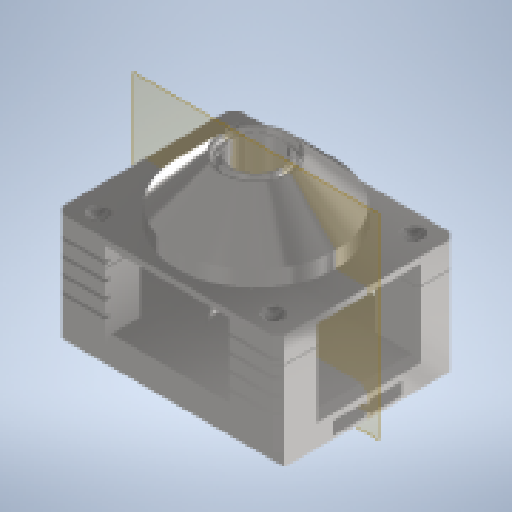
# Autodesk Inventor part: robotic-arm_base
Saved by Autodesk Inventor 2023 (Build 270158000, 158)
## iProperties
Created: 2023-11-19
Part Number: robotic-arm_base
Material: Steel, Mild
Document SubType Name: Modeling
Designer: Beatrice
Density: 7.85 g/cm^3
Appearance: Semi-Polished
Author: Beatrice
Autodesk Inventor part; units mm, degrees
ref_plane "YZ Plane" through (0, 0, 0) normal (1, 0, 0) x (0, 1, 0)
ref_plane "XZ Plane" through (0, 0, 0) normal (0, 1, 0) x (-1, 0, 0)
ref_plane "XY Plane" through (0, 0, 0) normal (0, 0, 1) x (1, 0, 0)
sketch "Sketch1" plane through (0, 0, 0) normal (1, 0, 0) x (0, 1, 0)
  line L0 (0, 25.2) -> (0, -4.2) construction
  line L1 (-30, 0) -> (5, 0) construction
  line L2 (0, 0) -> (-25, 0)
  line L3 (-25, 7) -> (-25, 0)
  line L4 (-7.6, 21) -> (-7.6, 6)
  line L5 (-7.6, 6) -> (0, 6)
  line L6 (0, 6) -> (0, 0)
  line L7 (-25, 7) -> (-11, 21)
  line L8 (-11, 21) -> (-7.6, 21)
  line L9 (-10.3, 21) -> (-8.3, 21)
  line L10 (-8.3, 21) -> (-8.3, 19)
  line L11 (-8.3, 19) -> (-10.3, 19)
  line L12 (-10.3, 19) -> (-10.3, 21)
  point P0 (-3.8, 6)
  point P1 (-9.3, 21)
  point P2 (-9.3, 19)
  dimension "d3" = 7.6
  dimension "d4" = 25
  dimension "d6" = 6
  dimension "d7" = 135
  dimension "d67" = 15
  dimension "d68" = 2
  constraints: 22 end point, 4 perpendicular, 3 midpoint, 3 point on line, 2 parallel, 1 collinear, 1 horizontal, 1 vertical alignment
  measures "d3" distance between parallel lines of L0 L4
  measures "d4" distance of L2.end L2.start
  measures "d6" distance between parallel lines of L5 L2
  measures "d7" angle of L3 L7
  measures "d67" vertical distance of point (-3.8, 6) point (-9.3, 21)
  measures "d68" distance of L10.end L11.end
revolve "Revolution1" add sketch "Sketch1" angle 360 about axis through (0, 0, 0) along (0, 0, -1)
sketch "Sketch2" plane through (0, 0, 0) normal (0, 0, -1) x (-1, 0, 0)
  line L0 (35.016, -28.0128) -> (-35.016, -28.0128)
  line L1 (-35.016, -28.0128) -> (-35.016, 28.0128)
  line L2 (-35.016, 28.0128) -> (35.016, 28.0128)
  line L3 (35.016, 28.0128) -> (35.016, -28.0128)
  line L4 (35.016, -28.0128) -> (-35.016, 28.0128) construction
  line L5 (-35.016, -28.0128) -> (35.016, 28.0128) construction
  circle A0 centre (0, 0) radius 25 projected
  line L6 (20.7481, -16.5984) -> (29.2519, -23.4016) construction
  line L7 (29.2519, -16.5984) -> (20.7481, -23.4016) construction
  circle A1 centre (-27.516, -22.0128) radius 3
  line L8 (49.0224, 0) -> (-49.0224, 0) construction
  line L9 (0, -39.2179) -> (0, 39.2179) construction
  circle A2 centre (-27.516, 22.0128) radius 3
  circle A3 centre (27.516, -22.0128) radius 3
  circle A4 centre (27.516, 22.0128) radius 3
  point P0 (25, -20)
  dimension "d9" = 6
  dimension "d10" = 6
  constraints: 16 end point, 4 centre point, 4 midpoint, 3 point on line, 3 symmetric about line, 2 parallel, 1 horizontal, 1 perpendicular, 3 other
  measures "d9" diameter of A1
  measures "d10" distance from line of L0 A1.centre
extrude "Extrusion1" add sketch "Sketch2" against normal blind 2
sketch "Sketch3" plane through (35.016, 28.0128, 0) normal (0, 0, -1) x (-1, 0, 0)
  circle A0 centre (35.016, -28.0128) radius 25 projected
  circle A1 centre (35.016, -28.0128) radius 11 projected
  circle A2 centre (35.016, -28.0128) radius 7.6 projected
  circle A3 centre (35.016, -28.0128) radius 5
  dimension "d13" = 10
  constraints: 1 centre point, 1 coincident
  measures "d13" diameter of A3
extrude "Extrusion2" cut sketch "Sketch3" against normal blind 7.5 contours A1 | A2 | A3
sketch "Sketch4" plane through (35.016, 28.0128, 0) normal (0, 0, -1) x (-1, 0, 0)
  circle A0 centre (35.016, -28.0128) radius 11 projected
  circle A1 centre (7.5, -50.0256) radius 3 projected
  circle A2 centre (7.5, -6) radius 3 projected
  circle A3 centre (62.532, -50.0256) radius 3 projected
  circle A4 centre (62.532, -6) radius 3 projected
  line L0 (70.032, 0) -> (0, 0) projected
  line L1 (0, 0) -> (0, -56.0256) projected
  line L2 (0, -56.0256) -> (70.032, -56.0256) projected
  line L3 (70.032, -56.0256) -> (70.032, 0) projected
extrude "Extrusion3" add sketch "Sketch4" along normal blind 30
sketch "Sketch5" plane through (-35.016, -28.0128, 2) normal (0, -1, 0) x (1, 0, 0)
  line L0 (24.016, -32) -> (24.016, 5.5) projected
  line L1 (10.5, 0) -> (10.5, -32) projected
  line L2 (4.5, 0) -> (4.5, -32) projected
  line L3 (46.016, -32) -> (46.016, 5.5) projected
  line L4 (59.532, 0) -> (59.532, -32) projected
  line L5 (65.532, 0) -> (65.532, -32) projected
  line L6 (70.032, 0) -> (70.032, -32) projected
  line L7 (0, 0) -> (70.032, 0) projected
  line L8 (0, 0) -> (0, -32) projected
  line L9 (70.032, -32) -> (0, -32) projected
  line L10 (15.5, -2) -> (54.532, -2)
  line L11 (54.532, -2) -> (54.532, -27)
  line L12 (54.532, -27) -> (15.5, -27)
  line L13 (15.5, -27) -> (15.5, -2)
  point P0 (35.016, -2)
  point P1 (35.016, -2)
  dimension "d18" = 5
  dimension "d19" = 5
  dimension "d20" = 25
  constraints: 8 end point, 2 parallel, 1 coincident, 1 horizontal, 1 midpoint, 1 perpendicular
  measures "d18" distance between parallel lines of L13 L1
  measures "d19" distance between parallel lines of L4 L11
  measures "d20" distance of L12.end L10.start
extrude "Extrusion4" cut sketch "Sketch5" against normal through all contours L12 L13 L10 L0 | L0 L10 L3 L12 | L3 L10 L11 L12
sketch "Sketch6" plane through (-35.016, -28.0128, 2) normal (-1, 0, 0) x (0, 0, 1)
  line L0 (0, 9) -> (-32, 9) projected
  line L1 (0, 9) -> (-32, 9) projected
  line L2 (0, 47.0256) -> (-32, 47.0256) projected
  line L3 (-2, 0) -> (-2, 56.0256) projected
  line L4 (-27, 0) -> (-27, 56.0256) projected
  line L5 (-2, 44) -> (-27, 44)
  line L6 (-27, 44) -> (-27, 13)
  line L7 (-27, 13) -> (-2, 13)
  line L8 (-2, 13) -> (-2, 44)
  point P0 (-2, 28.0128)
  point P1 (-2, 13)
  constraints: 8 end point, 2 parallel, 2 point on line, 1 horizontal, 1 perpendicular
extrude "Extrusion5" cut sketch "Sketch6" against normal through all contours L7 L4 L5 L3
sketch "Sketch7" plane through (-35.016, -28.0128, 2) normal (0, -1, 0) x (1, 0, 0)
  line L0 (15.5, -2) -> (15.5, -27) projected
  line L1 (0, -6) -> (15.5, -6)
  line L2 (15.5, -6) -> (15.5, -7)
  line L3 (15.5, -7) -> (0, -7)
  line L4 (0, -7) -> (0, -6)
  point P0 (35.016, -2)
  point P1 (15.5, -6)
  constraints: 8 end point, 2 parallel, 1 horizontal, 1 perpendicular, 1 point on line
extrude "Extrusion6" cut sketch "Sketch7" against normal blind 1.5
pattern_linear "Rectangular Pattern1" count 4 spacing 5 along (0, 0, -1) of "Extrusion6"
mirror "Mirror1" about plane through (0, 0, 0) normal (1, 0, 0) of "Extrusion6", "Rectangular Pattern1"
mirror "Mirror2" about plane through (0, 0, 0) normal (0, 1, 0) of "Extrusion6", "Rectangular Pattern1", "Mirror1"
chamfer "Chamfer1" distance 2 angle 45 4 edges at (35.016, -28.0128, -25) (35.016, 28.0128, -25) (-35.016, 28.0128, -25) (-35.016, -28.0128, -25)
chamfer "Chamfer2" distance 2 angle 45 4 edges at (0, -28.0128, -25) (35.016, 0.4872, -25) (0, 28.0128, -25) (-35.016, 0.4872, -25)
chamfer "Chamfer3" distance 2 angle 45 4 edges at (19.516, 15.9872, -12.5) (-19.516, -15.0128, -12.5) (-19.516, 15.9872, -12.5) (19.516, -15.0128, -12.5)
thread "Thread1" size "M6x1" class "6H" standard "ANSI Metric M Profile" full length
thread "Thread2" size "M6x1" class "6H" standard "ANSI Metric M Profile" full length
thread "Thread3" size "M6x1" class "6H" standard "ANSI Metric M Profile" full length
thread "Thread4" size "M6x1" class "6H" standard "ANSI Metric M Profile" full length
sketch "Sketch8" plane through (35.016, -26.0128, 2) normal (1, 0, 0) x (0, 0, -1)
  line L0 (7, 54.0256) -> (11, 54.0256) projected
  line L1 (8, -1.9744) -> (8.3, -1.9744)
  line L2 (8.3, -1.9744) -> (8.3, 54.0256)
  line L3 (8.3, 54.0256) -> (8, 54.0256)
  line L4 (8, 54.0256) -> (8, -1.9744)
  point P0 (2, 26.0128)
  dimension "d47" = 0.3
  dimension "d48" = 56
  constraints: 8 end point, 2 parallel, 1 horizontal, 1 perpendicular, 1 point on line
  measures "d47" distance of L3.end L2.end
  measures "d48" distance of L3.end L1.start
extrude "Extrusion7" cut sketch "Sketch8" against normal through all
sketch "Sketch9" plane through (35.016, 28.0128, -30) normal (0, 0, -1) x (-1, 0, 0)
  line L0 (0, -2) -> (0, -54.0256) projected
  line L1 (70.032, -54.0256) -> (68.032, -56.0256) projected
  line L2 (70.032, -54.0256) -> (70.032, -2) projected
  line L3 (68.032, 0) -> (70.032, -2) projected
  line L4 (68.032, 0) -> (2, 0) projected
  line L5 (0, -2) -> (2, 0) projected
  line L6 (0, -2) -> (0, -54.0256) projected
  line L7 (2, -56.0256) -> (0, -54.0256) projected
  line L8 (2, -56.0256) -> (68.032, -56.0256) projected
  circle A0 centre (62.532, -6) radius 3 projected
  circle A1 centre (62.532, -50.0256) radius 3 projected
  circle A2 centre (7.5, -6) radius 3 projected
  circle A3 centre (7.5, -50.0256) radius 3 projected
  circle A4 centre (35.016, -28.0128) radius 11 projected
extrude "Extrusion8" add sketch "Sketch9" against normal blind 3 contours A4
sketch "Sketch10" plane through (35.016, -26.0128, -30) normal (1, 0, 0) x (0, 0, -1)
  line L0 (-23.7, 11) -> (-23.7, 0) projected
  line L1 (0, 0) -> (-23.7, 0) projected
  line L2 (0, 52.0256) -> (0, 0) projected
  line L3 (-23.7, 52.0256) -> (0, 52.0256) projected
  line L4 (-23.7, 52.0256) -> (-23.7, 42) projected
  line L5 (-23.7, 42) -> (-3, 42) projected
  line L6 (-3, 11) -> (-3, 42) projected
  line L7 (-3, 11) -> (-23.7, 11) projected
  line L8 (-23.7, 0) -> (0, 0) projected
  line L9 (-3, 0) -> (5, 0)
  line L10 (5, 0) -> (5, 52)
  line L11 (5, 52) -> (-3, 52)
  line L12 (-3, 52) -> (-3, 0)
  line L13 (-1, 15.0128) -> (3, 15.0128)
  line L14 (3, 15.0128) -> (3, 37.0128)
  line L15 (3, 37.0128) -> (-1, 37.0128)
  line L16 (-1, 37.0128) -> (-1, 15.0128)
  line L17 (3, 25.5128) -> (2, 25.5128)
  line L18 (2, 25.5128) -> (2, 26.5128)
  line L19 (2, 26.5128) -> (3, 26.5128)
  line L20 (3, 26.5128) -> (3, 25.5128)
  line L21 (0, 0) -> (0, 52.0256) projected
  line L22 (-1, 25.5128) -> (0, 25.5128)
  line L23 (0, 25.5128) -> (0, 26.5128)
  line L24 (0, 26.5128) -> (-1, 26.5128)
  line L25 (-1, 26.5128) -> (-1, 25.5128)
  point P0 (-30, 26.0128)
  point P1 (-1, 26.0128)
  point P2 (2, 26.0128)
  point P3 (0, 26.0128)
  point P4 (2.5, 25.5128)
  point P5 (2.5, 26.5128)
  point P6 (1, 15.0128)
  point P7 (-1, 26.5128)
  point P8 (0, 26.5128)
  point P9 (0, 37.0128)
  point P10 (0, 25.5128)
  point P11 (0, 15.0128)
  point P12 (0, 52)
  point P13 (3, 26.5128)
  dimension "d54" = 22
  dimension "d57" = 11
  dimension "d58" = 1
  constraints: 32 end point, 8 parallel, 6 midpoint, 6 point on line, 4 horizontal, 4 perpendicular, 2 horizontal alignment
  measures "d54" distance of L13.end L14.end
  measures "d57" vertical distance of point (1, 15.013) point (2, 26.013)
  measures "d58" distance of point (2.5, 26.513) point (2.5, 25.513)
extrude "Extrusion9" cut sketch "Sketch10" against normal through all contours L13 L16 L22 L2 | L2 L24 L16 L15
extrude "Extrusion10" add sketch "Sketch10" against normal up to surface (70.032 mm away) contours L2 L13 L14 L15 L11 L10 L9 | L17 L18 L19 L14
fillet "Fillet1" radius 0.5 12 edges at (0, 11, -33) (0, -0.5, -33) (0, -11, -33) (0, 0.5, -33) (0, 0.5, -29) (-35.016, -5.75, -29) (0, 0.5, -30) (0, -0.5, -32) (0, -0.5, -30) (0, 0.5, -32) (0, -11, -29) (0, 11, -29)
chamfer "Chamfer4" distance 1 angle 45 9 edges at (35.016, 15.9872, -16.65) (35.016, -15.0128, -16.65) (35.016, 15.9872, -3) (35.016, -15.0128, -3) (0, -26.0128, -35) (35.016, -0.0128, -35) (-35.016, -15.0128, -16.65) (-35.016, -0.0128, -35) (0, 25.9872, -35)
revolve "Revolution2" cut sketch "Sketch1" angle 360 about axis through (0, 0, 0) along (0, 0, -1) contours L8 L10 L11 L12
fillet "Fillet2" radius 1 2 edges at (0, 10.3, 19) (0, 8.3, 19)
fillet "Fillet3" radius 0.2 4 edges at (0, 11, 21) (0, 10.3, 21) (0, 8.3, 21) (0, 7.6, 21)
ref_plane "Work Plane1" through (0, 26.0128, -6.3) normal (1, 0, 0) x (0, 0, -1)
body "Solid1"
